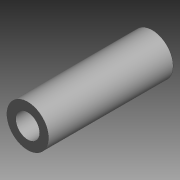
# Autodesk Inventor part: Linkage Mount
Saved by Autodesk Inventor 2014 SP1 (Build 180222100, 222)
## iProperties
Created: 2013-12-25
Part Number: Linkage Mount
Material: Generic
Document SubType Name: Modeling
Designer: tom
Density: 1 g/cm^3
Appearance: Default
Author: tom
Autodesk Inventor part; units mm, degrees
ref_plane "YZ Plane" through (0, 0, 0) normal (1, 0, 0) x (0, 1, 0)
ref_plane "XZ Plane" through (0, 0, 0) normal (0, 1, 0) x (-1, 0, 0)
ref_plane "XY Plane" through (0, 0, 0) normal (0, 0, 1) x (1, 0, 0)
sketch "Sketch1" plane through (0, 0, 0) normal (0, 0, 1) x (1, 0, 0)
  circle A0 centre (0, 0) radius 3.175
  circle A1 centre (0, 0) radius 1.825
  dimension "d0" = 6.35
  dimension "d1" = 3.65
  constraints: 2 centre point, 2 coincident
  measures "d0" diameter of A0
  measures "d1" diameter of A1
extrude "Extrusion1" add sketch "Sketch1" along normal blind 19
chamfer "Chamfer1" distance 0.5 angle 45 2 edges at (-1.825, 0, 19) (-1.825, 0, 0)
body "Solid1"
